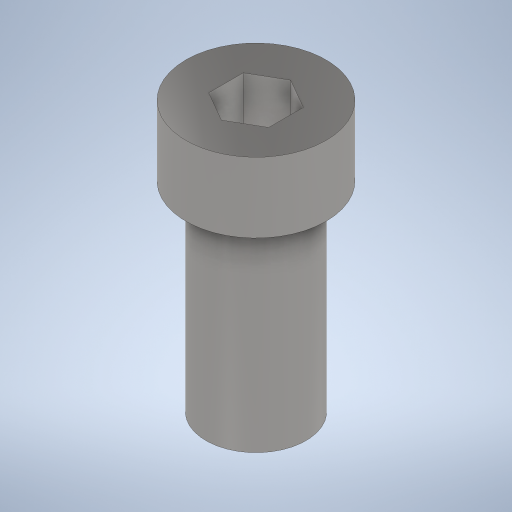
# Autodesk Inventor part: M5 x 10
Saved by Autodesk Inventor 2024.2 (Build 282272000, 272)
## iProperties
Created: 2024-01-31
Part Number: M5 x 10
Material: Stainless Steel
Document SubType Name: Modeling
Designer: jp.reyesf
Density: 8 g/cm^3
Appearance: Semi-Polished
Author: jp.reyesf
Autodesk Inventor part; units mm, degrees
ref_plane "YZ Plane" through (0, 0, 0) normal (1, 0, 0) x (0, 1, 0)
ref_plane "XZ Plane" through (0, 0, 0) normal (0, 1, 0) x (-1, 0, 0)
ref_plane "XY Plane" through (0, 0, 0) normal (0, 0, 1) x (1, 0, 0)
sketch "Sketch1" plane through (0, 0, 0) normal (0, 1, 0) x (-1, 0, 0)
  circle A0 centre (0, 0) radius 3.5
  circle A1 centre (0, 0) radius 2.5
  dimension "d0" = 7
  dimension "d1" = 5
  constraints: 2 centre point, 2 coincident
  measures "d0" diameter of A0
  measures "d1" diameter of A1
extrude "Extrusion1" add sketch "Sketch1" against normal blind 10 contours A1
extrude "Extrusion2" add sketch "Sketch1" along normal blind 3.5 contours A0 | A1
sketch "Sketch2" plane through (0, 3.5, 0) normal (0, 1, 0) x (1, 0, 0)
  circle A0 centre (0, 0) radius 2.5 projected
  line L0 (-1.5, -0.866) -> (-1.5, 0.866)
  line L1 (-1.5, 0.866) -> (0, 1.7321)
  line L2 (0, 1.7321) -> (1.5, 0.866)
  line L3 (1.5, 0.866) -> (1.5, -0.866)
  line L4 (1.5, -0.866) -> (0, -1.7321)
  line L5 (0, -1.7321) -> (-1.5, -0.866)
  dimension "d6" = 3
  constraints: 12 end point, 1 coincident, 1 vertical, 13 other
  measures "d6" distance between parallel lines of L3 L0
extrude "Extrusion3" cut sketch "Sketch2" against normal blind 2.5 contours L0 L1 L2 L3 L4 L5
equation "\"d0\" = D_"
equation "\"d1\" = M_"
equation "\"d2\" = L_"
equation "\"d4\" = K_"
equation "\"d6\" = S_"
equation "\"d7\" = t_"
equation "\"K_\" = 3.5"
equation "\"D_\" = 7"
equation "\"S_\" = 3"
equation "\"t_\" = 2.5"
equation "\"M_\" = 5"
equation "\"L_\" = 10"
body "Solid1"
